Autodesk Inventor part; units mm, degrees
(part 2 of 2)
  line L965 (4.8201, 11.9494) -> (5.2038, 11.1308)
  line L966 (5.2038, 11.1308) -> (5.6411, 10.3396)
  line L967 (5.6411, 10.3396) -> (6.13, 9.5793)
  line L968 (6.13, 9.5793) -> (6.6685, 8.8531)
  line L969 (6.6685, 8.8531) -> (7.2541, 8.1645)
  line L970 (7.2541, 8.1645) -> (7.8842, 7.5163)
  line L971 (7.8842, 7.5163) -> (8.5561, 6.9114)
  line L972 (8.5561, 6.9114) -> (9.2667, 6.3527)
  line L973 (9.2667, 6.3527) -> (10.013, 5.8424)
  line L974 (10.013, 5.8424) -> (10.7915, 5.3829)
  line L975 (10.7915, 5.3829) -> (11.5989, 4.9763)
  line L976 (11.5989, 4.9763) -> (12.4315, 4.6243)
  line L977 (12.4315, 4.6243) -> (13.2858, 4.3284)
  line L978 (13.2858, 4.3284) -> (14.1578, 4.0901)
  line L979 (14.1578, 4.0901) -> (15.0437, 3.9103)
  line L980 (15.0437, 3.9103) -> (15.9397, 3.7899)
  line L981 (15.9397, 3.7899) -> (16.8416, 3.7293)
  line L982 (16.8416, 3.7293) -> (17.7456, 3.7289)
  line L983 (17.7456, 3.7289) -> (18.6477, 3.7887)
  line L984 (18.6477, 3.7887) -> (19.5437, 3.9084)
  line L985 (19.5437, 3.9084) -> (20.4298, 4.0874)
  line L986 (20.4298, 4.0874) -> (21.302, 4.3249)
  line L987 (21.302, 4.3249) -> (22.1565, 4.62)
  line L988 (22.1565, 4.62) -> (22.9895, 4.9713)
  line L989 (22.9895, 4.9713) -> (23.7972, 5.3773)
  line L990 (23.7972, 5.3773) -> (23.9512, 6.0597)
  line L991 (23.9512, 6.0597) -> (18.3881, 13.9532)
  line L992 (18.3881, 13.9532) -> (17.5223, 14.2808)
  line L993 (17.5223, 14.2808) -> (17.0843, 14.2802)
  line L994 (17.0843, 14.2802) -> (16.6507, 14.3429)
  line L995 (16.6507, 14.3429) -> (16.2308, 14.4675)
  line L996 (16.2308, 14.4675) -> (15.8332, 14.6514)
  line L997 (15.8332, 14.6514) -> (15.4664, 14.8908)
  line L998 (15.4664, 14.8908) -> (15.1379, 15.1806)
  line L999 (15.1379, 15.1806) -> (14.8547, 15.5148)
  line L1000 (14.8547, 15.5148) -> (14.0444, 15.9625)
  line L1001 (20.085, 15.1491) -> (25.648, 7.2556)
  line L1002 (25.648, 7.2556) -> (26.3425, 7.1711)
  line L1003 (26.3425, 7.1711) -> (26.9964, 7.7953)
  line L1004 (26.9964, 7.7953) -> (27.6074, 8.4616)
  line L1005 (27.6074, 8.4616) -> (28.1726, 9.1671)
  line L1006 (28.1726, 9.1671) -> (28.6897, 9.9086)
  line L1007 (28.6897, 9.9086) -> (29.1562, 10.683)
  line L1008 (29.1562, 10.683) -> (29.5702, 11.4866)
  line L1009 (29.5702, 11.4866) -> (29.9298, 12.316)
  line L1010 (29.9298, 12.316) -> (30.2335, 13.1675)
  line L1011 (30.2335, 13.1675) -> (30.4798, 14.0373)
  line L1012 (30.4798, 14.0373) -> (30.6676, 14.9216)
  line L1013 (30.6676, 14.9216) -> (30.7962, 15.8164)
  line L1014 (30.7962, 15.8164) -> (30.865, 16.7177)
  line L1015 (30.865, 16.7177) -> (30.8737, 17.6217)
  line L1016 (30.8737, 17.6217) -> (30.8221, 18.5242)
  line L1017 (30.8221, 18.5242) -> (30.7107, 19.4214)
  line L1018 (30.7107, 19.4214) -> (30.5398, 20.3091)
  line L1019 (30.5398, 20.3091) -> (30.3101, 21.1834)
  line L1020 (30.3101, 21.1834) -> (30.0229, 22.0405)
  line L1021 (30.0229, 22.0405) -> (29.6792, 22.8767)
  line L1022 (29.6792, 22.8767) -> (29.2806, 23.6881)
  line L1023 (29.2806, 23.6881) -> (28.829, 24.4712)
  line L1024 (28.829, 24.4712) -> (28.3262, 25.2225)
  line L1025 (28.3262, 25.2225) -> (27.7746, 25.9386)
  line L1026 (27.7746, 25.9386) -> (27.1765, 26.6165)
  line L1027 (27.1765, 26.6165) -> (26.5346, 27.2531)
  line L1028 (26.5346, 27.2531) -> (25.8518, 27.8456)
  line L1029 (25.8518, 27.8456) -> (25.1311, 28.3913)
  line L1030 (25.1311, 28.3913) -> (24.3757, 28.8878)
  line L1031 (24.3757, 28.8878) -> (23.7077, 28.6799)
  line L1032 (23.7077, 28.6799) -> (19.6533, 19.9155)
  line L1033 (19.6533, 19.9155) -> (19.8025, 19.0018)
  line L1034 (19.8025, 19.0018) -> (20.022, 18.6228)
  line L1035 (20.022, 18.6228) -> (20.1845, 18.216)
  line L1036 (20.1845, 18.216) -> (20.2865, 17.79)
  line L1037 (20.2865, 17.79) -> (20.326, 17.3537)
  line L1038 (20.326, 17.3537) -> (20.3022, 16.9163)
  line L1039 (20.3022, 16.9163) -> (20.2154, 16.487)
  line L1040 (20.2154, 16.487) -> (20.0676, 16.0746)
  line L1041 (20.0676, 16.0746) -> (20.085, 15.1491)
  line L1042 (17.7692, 20.7871) -> (21.8236, 29.5515)
  line L1043 (21.8236, 29.5515) -> (21.5495, 30.1952)
  line L1044 (21.5495, 30.1952) -> (20.682, 30.4494)
  line L1045 (20.682, 30.4494) -> (19.7995, 30.6454)
  line L1046 (19.7995, 30.6454) -> (18.9059, 30.7821)
  line L1047 (18.9059, 30.7821) -> (18.0052, 30.8591)
  line L1048 (18.0052, 30.8591) -> (17.1013, 30.876)
  line L1049 (17.1013, 30.876) -> (16.1984, 30.8327)
  line L1050 (16.1984, 30.8327) -> (15.3003, 30.7295)
  line L1051 (15.3003, 30.7295) -> (14.4111, 30.5667)
  line L1052 (14.4111, 30.5667) -> (13.5346, 30.3451)
  line L1053 (13.5346, 30.3451) -> (12.6749, 30.0656)
  line L1054 (12.6749, 30.0656) -> (11.8357, 29.7296)
  line L1055 (11.8357, 29.7296) -> (11.0207, 29.3385)
  line L1056 (11.0207, 29.3385) -> (10.2335, 28.894)
  line L1057 (10.2335, 28.894) -> (9.4776, 28.3981)
  line L1058 (9.4776, 28.3981) -> (8.7564, 27.853)
  line L1059 (8.7564, 27.853) -> (8.0731, 27.2611)
  line L1060 (8.0731, 27.2611) -> (7.4307, 26.6251)
  line L1061 (7.4307, 26.6251) -> (6.832, 25.9478)
  line L1062 (6.832, 25.9478) -> (6.2798, 25.2321)
  line L1063 (6.2798, 25.2321) -> (5.7763, 24.4812)
  line L1064 (5.7763, 24.4812) -> (5.324, 23.6985)
  line L1065 (5.324, 23.6985) -> (4.9248, 22.8875)
  line L1066 (4.9248, 22.8875) -> (4.5803, 22.0516)
  line L1067 (4.5803, 22.0516) -> (4.2923, 21.1947)
  line L1068 (4.2923, 21.1947) -> (4.062, 20.3206)
  line L1069 (4.062, 20.3206) -> (3.8903, 19.433)
  line L1070 (3.8903, 19.433) -> (3.778, 18.536)
  line L1071 (3.778, 18.536) -> (3.7257, 17.6335)
  line L1072 (3.7257, 17.6335) -> (4.2398, 17.159)
  line L1073 (4.2398, 17.159) -> (13.8572, 18.03)
  line L1074 (13.8572, 18.03) -> (14.5738, 18.616)
  line L1075 (14.5738, 18.616) -> (14.7924, 18.9956)
  line L1076 (14.7924, 18.9956) -> (15.0634, 19.3397)
  line L1077 (15.0634, 19.3397) -> (15.3813, 19.6411)
  line L1078 (15.3813, 19.6411) -> (15.7394, 19.8935)
  line L1079 (15.7394, 19.8935) -> (16.1301, 20.0915)
  line L1080 (16.1301, 20.0915) -> (16.5453, 20.2311)
  line L1081 (16.5453, 20.2311) -> (16.9763, 20.3092)
  line L1082 (16.9763, 20.3092) -> (17.7692, 20.7871)
  circle A0 centre (17.2995, 17.2995) radius 0.5
  line L1083 (11.533, 17.2995) -> (23.0661, 17.2995)
  line L1084 (17.2995, 11.533) -> (17.2995, 23.0661)
  point P0 (0, 0)
  point P1 (0.1047, 15.3995)
  constraints: 2170 end point, 1 centre point
extrude "Выдавливание1" add sketch "Эскиз1" along normal blind 5
